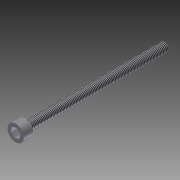
# Autodesk Inventor part: Bolt BD Drill motor mount
Saved by Autodesk Inventor 2012 (Build 160160000, 160)
## iProperties
Created: 2012-06-30
Part Number: Bolt BD Drill motor mount
Material: Default
Document SubType Name: Modeling
Designer: Bruce
Density: 1 g/cm^3
Author: Bruce
Autodesk Inventor part; units mm, degrees
ref_plane "YZ Plane" through (0, 0, 0) normal (1, 0, 0) x (0, 1, 0)
ref_plane "XZ Plane" through (0, 0, 0) normal (0, 1, 0) x (-1, 0, 0)
ref_plane "XY Plane" through (0, 0, 0) normal (0, 0, 1) x (1, 0, 0)
sketch "Sketch1" plane through (0, 0, 0) normal (0, 0, 1) x (1, 0, 0)
  circle A0 centre (0, 0) radius 4.445
  circle A1 centre (0, 0) radius 2.413
  line L0 (0.6651, 2.673) -> (2.6474, 0.7606)
  line L1 (2.6474, 0.7606) -> (1.9824, -1.9125)
  line L2 (1.9824, -1.9125) -> (-0.6651, -2.673)
  line L3 (-0.6651, -2.673) -> (-2.6474, -0.7606)
  line L4 (-2.6474, -0.7606) -> (-1.9824, 1.9125)
  line L5 (-1.9824, 1.9125) -> (0.6651, 2.673)
  dimension "d0" = 4.826
  dimension "d1" = 8.89
  constraints: 12 end point, 3 coincident, 2 centre point, 13 other
  measures "d0" diameter of A1
  measures "d1" diameter of A0
extrude "Extrusion1" add sketch "Sketch1" against normal blind 76.2 contours A1 L1 L2 L3 L4 L5 L0 | L0 A1 | A1 L1 | L5 A1 | A1 L2 | L4 A1 | A1 L3
extrude "Extrusion2" add sketch "Sketch1" along normal blind 5.08
thread "Thread1" size "10-32 UNF" class "2A" standard "ANSI Unified Screw Threads" full length
body "Solid1"
